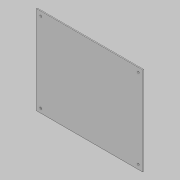
# Autodesk Inventor part: front_panel
Saved by Autodesk Inventor 2021.2 (Build 252289000, 289)
## iProperties
Created: 2021-08-04
Part Number: front_panel
Material: Generic
Document SubType Name: Modeling
Designer: gisen
Density: 1 g/cm^3
Appearance: Default
Author: gisen
Autodesk Inventor part; units mm, degrees
ref_plane "YZ Plane" through (0, 0, 0) normal (1, 0, 0) x (0, 1, 0)
ref_plane "XZ Plane" through (0, 0, 0) normal (0, 1, 0) x (-1, 0, 0)
ref_plane "XY Plane" through (0, 0, 0) normal (0, 0, 1) x (1, 0, 0)
sketch "スケッチ2" plane through (0, 0, 0) normal (0, 0, 1) x (1, 0, 0)
  line L0 (180, 150) -> (-180, 150)
  line L1 (-180, 150) -> (-180, -150)
  line L2 (-180, -150) -> (180, -150)
  line L3 (180, -150) -> (180, 150)
  line L4 (180, 150) -> (-180, -150) construction
  line L5 (-180, 150) -> (180, -150) construction
  point P0 (0, 0)
  dimension "d0" = 360
  dimension "d1" = 300
  constraints: 12 end point, 2 midpoint, 2 parallel, 1 horizontal, 1 perpendicular
  measures "d0" distance of L2.end L1.end
  measures "d1" distance of L1.end L0.end
extrude "押し出し1" add sketch "スケッチ2" along normal blind 3
sketch "スケッチ3" plane through (0, 0, 3) normal (0, 0, 1) x (1, 0, 0)
  line L0 (-180, 150) -> (-180, -150) construction
  line L1 (-180, -150) -> (180, -150) construction
  line L2 (180, -150) -> (180, 150) construction
  line L3 (180, 150) -> (-180, 150) construction
  line L4 (165, 135) -> (-165, 135) construction
  line L5 (-165, 135) -> (-165, -135) construction
  line L6 (-165, -135) -> (165, -135) construction
  line L7 (165, -135) -> (165, 135) construction
  line L8 (165, 135) -> (-165, -135) construction
  line L9 (-165, 135) -> (165, -135) construction
  point P0 (0, 0)
  dimension "d4" = 15
  dimension "d5" = 15
  constraints: 12 end point, 2 midpoint, 2 parallel, 1 horizontal, 1 perpendicular
  measures "d4" distance between parallel lines of L0 L5
  measures "d5" distance between parallel lines of L3 L4
hole "穴1" at (-165, 135, 3) at (165, 135, 3) at (165, -135, 3) at (-165, -135, 3) direction (0, 0, -1) diameter 6.6 end through all
equation "\"d5\" = d4"
